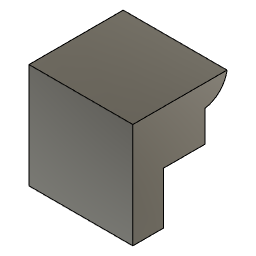
Jack 3D model v2 (Autodesk Fusion 360 design; units mm, degrees)
Autodesk Fusion 360 part; units mm, degrees
sketch "Sketch1" plane through (0, 0, 0) normal (1, 0, 0) x (0, 1, 0)
  line L0 (-75, 38.1238) -> (-29.6248, 38.1238)
  line L1 (-29.6248, 38.1238) -> (-14.6248, 38.1238) construction
  line L2 (-40.2314, 27.5172) -> (-40.2314, 12.5172)
  line L3 (-40.2314, 12.5172) -> (-60.2314, 12.5172)
  line L4 (-60.2314, 12.5172) -> (-60.2314, -12.4828)
  line L5 (-75, 38.1238) -> (-75, -12.4828)
  arc A0 (-40.2314, 27.5172) -> (-29.6248, 38.1238) centre (-42.1008, 39.9932) ccw
  line L6 (-60.2314, -12.4828) -> (-75, -12.4828)
  dimension "d4" = 15
  dimension "d5" = 15
  dimension "d6" = 20
  dimension "d7" = 25
  constraint horizontal L0
  constraint horizontal L1
  constraint perpendicular L0 L2
  constraint perpendicular L2 L3
  constraint perpendicular L3 L4
  constraint perpendicular L5 L6
  measures "d4" distance of L0.end L2.start
  measures "d5" distance of L2.start L2.end
  measures "d6" distance of L2.end L3.end
  measures "d7" distance of L3.end L4.end
extrude "Extrude1" add sketch "Sketch1" along normal blind 50
